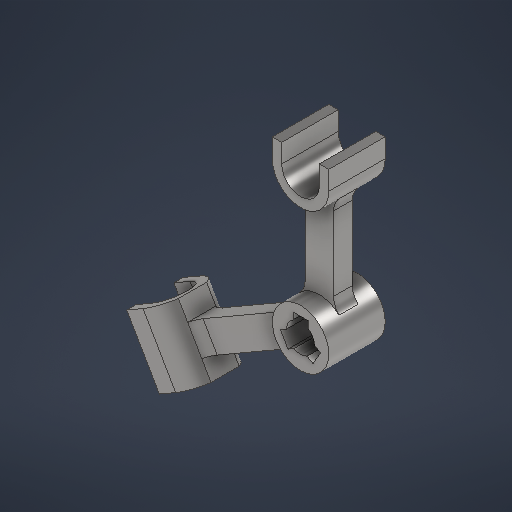
# Autodesk Inventor part: Pieza16
Saved by Autodesk Inventor 2026.2 (Build 302298000, 298)
## iProperties
Created: 2025-12-24
Part Number: Pieza16
Material: Acero inoxidable
Document SubType Name: Modeling
Designer: vicho
Mass: 387.716 g
Surface Area: 199.123 cm^2
Volume: 48.4645 cm^3
Density: 8 g/cm^3
Appearance: Semipulido
Author: vicho
Autodesk Inventor part; units mm, degrees
ref_plane "YZ Plane" through (0, 0, 0) normal (1, 0, 0) x (0, 1, 0)
ref_plane "XZ Plane" through (0, 0, 0) normal (0, 1, 0) x (-1, 0, 0)
ref_plane "XY Plane" through (0, 0, 0) normal (0, 0, 1) x (1, 0, 0)
sketch "Boceto1" plane through (0, 0, 0) normal (0, 0, 1) x (1, 0, 0)
  line L0 (0, 75) -> (0, -75) construction
  line L1 (-206.9145, 0) -> (206.9145, 0) construction
  line L2 (-7.5, 62.0096) -> (-7.5, 12.9904)
  line L3 (7.5, 62.0096) -> (7.5, 12.9904)
  circle A0 centre (0, 0) radius 15
  line L4 (-15, 0) -> (-67.4917, -30.3061)
  line L5 (-7.5, -12.9904) -> (-59.9917, -43.2965)
  line L6 (-15, 85) -> (-15, 75)
  line L7 (15, 85.0608) -> (15, 75)
  arc A1 (-10, 75.0296) -> (9.9998, 75.0608) centre (0, 75) ccw
  line L8 (-10, 75.0296) -> (-10, 85)
  line L9 (-10, 85) -> (-15, 85)
  line L10 (15, 85.0608) -> (9.9998, 85.0608)
  line L11 (9.9998, 85.0608) -> (9.9998, 75.0608)
  arc A2 (-15, 75) -> (-7.5, 62.0096) centre (0, 75) ccw
  arc A3 (7.5, 62.0096) -> (15, 75) centre (0, 75) ccw
  line L12 (4, 10) -> (-4, 10)
  line L13 (-4, 10) -> (-4, 6.3443)
  line L14 (4, 10) -> (4, 6.3443)
  line L15 (-10.6603, -1.5359) -> (-6.6603, -8.4641)
  line L16 (-6.6603, -8.4641) -> (-3.4943, -6.6362)
  line L17 (-10.6603, -1.5359) -> (-7.4943, 0.292)
  line L18 (6.6603, -8.4641) -> (10.6603, -1.5359)
  line L19 (10.6603, -1.5359) -> (7.4943, 0.292)
  line L20 (6.6603, -8.4641) -> (3.4943, -6.6362)
  arc A4 (-4, 6.3443) -> (-7.5, 0) centre (0, 0) ccw
  arc A5 (-3.4943, -6.6362) -> (3.4943, -6.6362) centre (0, 0) ccw
  arc A6 (7.5, 0) -> (4, 6.3443) centre (0, 0) ccw
  line L21 (0, 0) -> (-75, -43.3013) construction
  line L22 (-72.4019, -21.8013) -> (-92.3205, -33.3013)
  line L23 (-92.3205, -33.3013) -> (-75, -63.3013)
  line L24 (-75, -63.3013) -> (-55.0814, -51.8013)
  line L25 (-55.0814, -51.8013) -> (-72.4019, -21.8013)
  arc A7 (-7.5, 62.0096) -> (7.5, 62.0096) centre (0, 75) ccw
  point P0 (7.5, 37.5)
  point P1 (15, 80.0304)
  point P2 (9.9998, 80.0608)
  dimension "d0" = 75
  dimension "d1" = 15
  dimension "d2" = 30
  dimension "d3" = 10
  dimension "d4" = 10
  dimension "d5" = 10
  dimension "d6" = 5
  dimension "d7" = 5.0002
  dimension "d8" = 30
  dimension "d10" = 10
  dimension "d11" = 8
  dimension "d14" = 360
  dimension "d16" = 15
  dimension "d17" = 120
  dimension "d19" = 75
  dimension "d20" = 30
  dimension "d21" = 10
  dimension "d22" = 13
  dimension "d23" = 191.9145
  constraints: 53 end point, 18 point on circle, 8 centre point, 7 coincident, 7 midpoint, 6 vertical, 5 perpendicular, 4 parallel, 4 point on line, 3 horizontal, 3 tangent, 2 symmetric about line, 27 other
  measures "d0" distance of point (0, 0) point (0, 75)
  measures "d1" distance from line of point (7.5, 37.5) L2
  measures "d2" distance between parallel lines of L7 L6
  measures "d3" radius of A1
  measures "d4" vertical distance of L6.start L0.start
  measures "d5" vertical distance of L11.end L7.start
  measures "d6" distance of L8.end L6.start
  measures "d7" horizontal distance of point (15, 80.03) point (10, 80.061)
  measures "d8" diameter of A0
  measures "d10" vertical distance of L12.end L21.start
  measures "d11" distance of L12.start L12.end
  measures "d16" distance between parallel lines of L5 L4
  measures "d17" angle of L21 L0
  measures "d19" horizontal distance of point (0, 0) L21.end
  measures "d20" vertical distance of L23.end L22.end
  measures "d21" distance from line of L21.end L23
  measures "d22" distance from line of L25 L21.end
  measures "d23" distance from line of L1.end L7
extrude "Extrusión1" add sketch "Boceto1" along normal mid plane 30 contours A2 L6 L9 L8 A1 L11 L10 L7 A3 A7 | A0 | L25 L24 L23 L22
extrude "Extrusión2" add sketch "Boceto1" along normal mid plane 10 contours A7 L3 A0 L2 | A0 L5 L25 L4
sketch "Boceto2" plane through (-92.3205, -33.3013, 15) normal (-0.5, 0.8660254, 0) x (0.8660254, 0.5, 0)
  line L0 (0, 30) -> (0, 0) construction
  line L1 (52.4312, 15) -> (-24.455, 15) construction
  arc A0 (10, 5) -> (10, 25) centre (10, 15) ccw
  line L2 (10, 25) -> (0, 25)
  line L3 (10, 5) -> (0, 5)
  line L4 (0, 25) -> (0, 5)
  line L5 (0, 30) -> (0, 0) projected
  line L6 (0, 0) -> (23, 0) projected
  arc A1 (10, 0) -> (10, 30) centre (10, 15) ccw
  line L7 (23, 30) -> (0, 30) projected
  line L8 (10, 30) -> (23, 30)
  line L9 (23, 30) -> (23, 22.4833)
  line L10 (23, 0) -> (23, 30) projected
  line L11 (23, 7.5167) -> (23, 0)
  line L12 (0, 30) -> (23, 30) projected
  point P0 (96.6025, 15)
  dimension "d28" = 10
  dimension "d29" = 10
  constraints: 14 end point, 6 point on circle, 6 point on line, 4 horizontal, 3 tangent, 2 centre point, 2 coincident, 2 collinear, 1 perpendicular
  measures "d28" distance from line of L0 point (10, 15)
  measures "d29" radius of A0
extrude "Extrusión3" cut sketch "Boceto2" against normal blind 50 contours L3 L4 L2 A0 | A1 L10 L6 | L7 L9 A1
fillet "Empalme1" radius 10 8 edges at (-63.7417, -36.8013, 5) (-63.7417, -36.8013, -5) (-15, 0, 0) (-7.5, 12.9904, 0) (-7.5, -12.9904, 0) (7.5, 12.9904, 0) (7.5, 62.0096, 0) (-7.5, 62.0096, 0)
